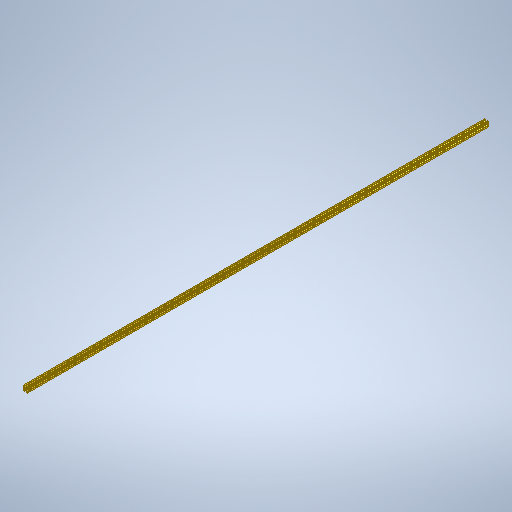
# Autodesk Inventor part: 20×20 4 slots profile_AST02002004
Saved by Autodesk Inventor 2025.2 (Build 292293000, 293)
## iProperties
Created: 2025-03-25
Part Number: 20×20 4 slots profile_AST02002004
Material: Ouro
Document SubType Name: Modeling
Designer: lucas
Density: 19.3 g/cm^3
Appearance: Metal quente 2400F
Author: lucas
Autodesk Inventor part; units mm, degrees
ref_plane "YZ Plane" through (0, 0, 0) normal (1, 0, 0) x (0, 1, 0)
ref_plane "XZ Plane" through (0, 0, 0) normal (0, 1, 0) x (-1, 0, 0)
ref_plane "XY Plane" through (0, 0, 0) normal (0, 0, 1) x (1, 0, 0)
sketch "Esboço1" plane through (0, 0, 0) normal (0, 0, 1) x (1, 0, 0)
  line L0 (-10, 10) -> (10, 10) construction
  circle A0 centre (0, 0) radius 2.5 construction
  line L1 (-4, 4) -> (4, 4) construction
  line L2 (0, 0) -> (-10, 10) construction
  line L3 (-6.5858, 8) -> (-4, 8) construction
  line L4 (-4, 8) -> (-4, 10) construction
  line L5 (-4, 10) -> (-10, 10) construction
  line L6 (-4, 4) -> (-4, -4) construction
  line L7 (-6.5858, 8) -> (-2.5858, 4) construction
  line L8 (-8, 6.5858) -> (-4, 2.5858) construction
  line L9 (-10, 10) -> (-10, 0) construction
  line L10 (-10, 10) -> (-10, 4) construction
  line L11 (-8, 6.5858) -> (-8, 4) construction
  line L12 (-8, 4) -> (-10, 4) construction
  line L13 (-10, 4) -> (-9.5, 4) construction
  line L14 (-9.5, 4) -> (-9.5, 4.5)
  line L15 (-9.5, 4.5) -> (-10, 4.5)
  line L16 (-10, 4.5) -> (-10, 4) construction
  line L17 (-10, 10) -> (-10, 4.5) construction
  line L18 (-9.5, 4) -> (-8, 4)
  line L19 (-4, 10) -> (-4.5, 10) construction
  line L20 (-4.5, 10) -> (-4.5, 9.5)
  line L21 (-4.5, 9.5) -> (-4, 9.5)
  line L22 (-4, 9.5) -> (-4, 10) construction
  line L23 (-4, 9.5) -> (-4, 8)
  line L24 (-4.5, 10) -> (-10, 10) construction
  arc A1 (-9.5, 10) -> (-10, 9.5) centre (-9.5, 9.5) ccw
  line L25 (-4.5, 10) -> (-9.5, 10)
  line L26 (-10, 9.5) -> (-10, 4.5)
  line L27 (-2.5858, 4) -> (0, 4) construction
  arc A2 (-5.3787, 8) -> (-5.7322, 7.1464) centre (-5.3787, 7.5) ccw
  line L28 (-5.3787, 8) -> (-4, 8)
  line L29 (-5.7322, 7.1464) -> (-2.5858, 4) construction
  arc A3 (-7.1464, 5.7322) -> (-8, 5.3787) centre (-7.5, 5.3787) ccw
  line L30 (-7.1464, 5.7322) -> (-4, 2.5858) construction
  line L31 (-8, 5.3787) -> (-8, 4)
  arc A4 (0, 2.5) -> (-2.5, 0) centre (0, 0) ccw
  line L32 (0, 4) -> (0, 2.5)
  line L33 (-4, 2.5858) -> (-4, 0) construction
  line L34 (-4, 0) -> (-2.5, 0)
  arc A5 (-2.7322, 4.1464) -> (-2.3787, 4) centre (-2.3787, 4.5) ccw
  line L35 (-5.7322, 7.1464) -> (-2.7322, 4.1464)
  line L36 (-2.3787, 4) -> (0, 4)
  arc A6 (-4, 2.3787) -> (-4.1464, 2.7322) centre (-4.5, 2.3787) ccw
  line L37 (-7.1464, 5.7322) -> (-4.1464, 2.7322)
  line L38 (-4, 2.3787) -> (-4, 0)
  point P0 (0, 10)
  point P1 (-3.25, 0)
  dimension "d0" = 20
  dimension "d2" = 5
  dimension "d3" = 6
  dimension "d5" = 2
  dimension "d7" = 1
  dimension "d8" = 6
  dimension "d9" = 1
  dimension "d10" = 0.5
  dimension "d11" = 0.5
  dimension "d12" = 0.5
  dimension "d14" = 0.5
  dimension "d15" = 0.5
  dimension "d16" = 10
  dimension "d17" = 2.5
  dimension "d20" = 0.5
  dimension "d21" = 0.5
  constraints: 78 end point, 16 point on line, 15 collinear, 14 point on circle, 13 tangent, 7 centre point, 6 parallel, 6 perpendicular, 5 horizontal, 4 midpoint, 3 equal length, 3 vertical, 3 vertical alignment, 2 horizontal alignment, 1 coincident
  measures "d0" distance of L0.start L0.end
  measures "d2" diameter of A0
  measures "d3" distance between parallel lines of L0 L1
  measures "d5" distance between parallel lines of L0 L3
  measures "d7" distance between parallel lines of L2 L7
  measures "d8" distance of L0.start L10.end
  measures "d9" distance between parallel lines of L8 L2
  measures "d10" distance of L15.end L14.end
  measures "d11" distance of L19.end L20.end
  measures "d12" radius of A1
  measures "d14" radius of A2
  measures "d15" radius of A3
  measures "d16" distance from line of point (0, 0) L0
  measures "d17" radius of A4
  measures "d20" radius of A5
  measures "d21" radius of A6
extrude "Extrusão1" add sketch "Esboço1" along normal mid plane 2000
mirror "Espelhar1" about plane through (0, 0, 0) normal (1, 0, 0) of "Extrusão1"
mirror "Espelhar2" about plane through (0, 0, 0) normal (0, 1, 0) of "Extrusão1", "Espelhar1"
equation "\"d16\" = 0.5 * d0"
